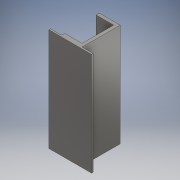
# Autodesk Inventor part: EE Track
Saved by Autodesk Inventor 2017 (Build 210142000, 142)
## iProperties
Created: 2018-10-18
Part Number: EE Track
Material: Generic
Document SubType Name: Modeling
Designer: Cameron
Density: 1 g/cm^3
Appearance: Galvanized
Author: Cameron
Autodesk Inventor part; units mm, degrees
ref_plane "YZ Plane" through (0, 0, 0) normal (1, 0, 0) x (0, 1, 0)
ref_plane "XZ Plane" through (0, 0, 0) normal (0, 1, 0) x (-1, 0, 0)
ref_plane "XY Plane" through (0, 0, 0) normal (0, 0, 1) x (1, 0, 0)
sketch "Sketch1" plane through (0, 0, 0) normal (0, 1, 0) x (-1, 0, 0)
  line L0 (0, 0) -> (27, 0)
  line L1 (27, 0) -> (27, -65)
  line L2 (27, -65) -> (0, -65)
  line L3 (0, -65) -> (0, 0)
  dimension "d0" = 27
  dimension "d1" = 65
  constraints: 8 end point, 2 parallel, 1 horizontal, 1 perpendicular
  measures "d0" distance of L1.end L2.end
  measures "d1" distance of L0.end L1.end
extrude "Extrusion1" add sketch "Sketch1" along normal blind 1
sketch "Sketch2" plane through (0, 1, 0) normal (0, 1, 0) x (1, 0, 0)
  line L0 (-27, 0) -> (0, 0) projected
  line L1 (0, 65) -> (-27, 65) projected
  line L2 (-13.5, 0) -> (-20, 0)
  line L3 (-20, 0) -> (-7, 0)
  line L4 (-7, 0) -> (-7, 65)
  line L5 (-20, 0) -> (-20, 65)
  line L6 (-7, 65) -> (-20, 65)
  dimension "d4" = 6.5
  dimension "d5" = 13
  constraints: 10 end point, 4 point on line, 3 perpendicular, 1 midpoint
  measures "d4" distance of L2.start L2.end
  measures "d5" distance of L2.end L3.end
extrude "Extrusion2" add sketch "Sketch2" along normal blind 2
sketch "Sketch3" plane through (0, 3, 0) normal (0, 1, 0) x (1, 0, 0)
  line L0 (-7, 0) -> (-7, 65) projected
  line L1 (-7, 65) -> (-20, 65) projected
  line L2 (-7, 0) -> (-9, 0)
  line L3 (-9, 0) -> (-9, 65)
  line L4 (-9, 65) -> (-7, 65)
  line L5 (-7, 65) -> (-7, 0)
  point P0 (0, 0)
  dimension "d8" = 2
  constraints: 8 end point, 2 parallel, 1 horizontal, 1 perpendicular, 1 point on line
  measures "d8" distance of L3.end L4.end
extrude "Extrusion3" add sketch "Sketch3" along normal blind 20
sketch "Sketch4" plane through (0, 23, 0) normal (0, 1, 0) x (1, 0, 0)
  line L0 (-20, 0) -> (-20, 65) projected
  line L1 (-7, 0) -> (-20, 0)
  line L2 (-20, 0) -> (-20, 65)
  line L3 (-20, 65) -> (-7, 65)
  line L4 (-7, 65) -> (-7, 0)
  point P0 (0, 0)
  constraints: 8 end point, 2 parallel, 1 horizontal, 1 perpendicular
extrude "Extrusion4" add sketch "Sketch4" along normal blind 2
body "Solid1"
